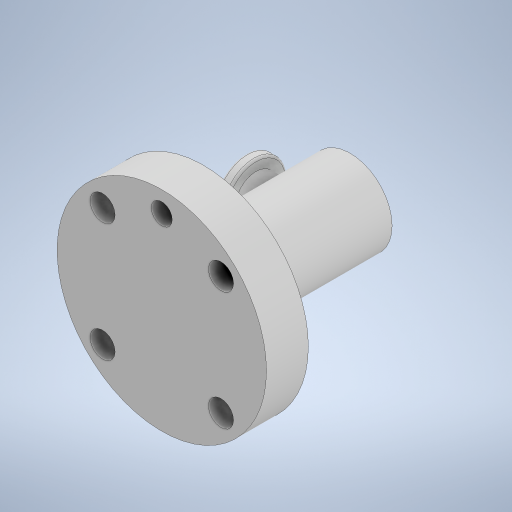
# Autodesk Inventor part: ACOPLE
Saved by Autodesk Inventor 2024 (Build 280153000, 153)
## iProperties
Created: 2023-05-11
Part Number: ACOPLE
Material: Genérico
Document SubType Name: Modeling
Designer: sebas
Density: 1 g/cm^3
Appearance: Valor por defecto
Author: sebas
Autodesk Inventor part; units mm, degrees
ref_plane "YZ Plane" through (0, 0, 0) normal (1, 0, 0) x (0, 1, 0)
ref_plane "XZ Plane" through (0, 0, 0) normal (0, 1, 0) x (-1, 0, 0)
sketch "Boceto4" plane through (0, 0, 0) normal (0, 0, 1) x (1, 0, 0)
  circle A0 centre (0, 0) radius 10
  circle A1 centre (0, 0) radius 7.582
  dimension "d6" = 20
  dimension "d7" = 15.164
  constraints: 2 centre point, 2 coincident
  measures "d6" diameter of A0
  measures "d7" diameter of A1
extrude "Extrusión3" add sketch "Boceto4" along normal blind 40
sketch "Boceto5" plane through (0, 0, 40) normal (0, 0, 1) x (1, 0, 0)
  circle A0 centre (0, 0) radius 7.582
  constraints: 1 centre point, 1 coincident
extrude "Extrusión4" add sketch "Boceto5" against normal blind 25
ref_plane "Plano de trabajo2" through (-10, 0, 0) normal (1, 0, 0) x (0, 1, 0)
sketch "Boceto6" plane through (-10, 0, 0) normal (1, 0, 0) x (0, 1, 0)
  line L0 (0, 0) -> (0, 10)
  circle A0 centre (0, 10) radius 5
  dimension "d14" = 10
  dimension "d15" = 10
  constraints: 2 end point, 1 centre point, 1 coincident, 1 vertical
  measures "d14" distance of L0.start L0.end
  measures "d15" diameter of A0
extrude "Extrusión5" cut sketch "Boceto6" along normal blind 10
ref_plane "Plano de trabajo3" through (-15, 0, 0) normal (1, 0, 0) x (0, 1, 0)
sketch "Boceto8" plane through (-15, 0, 0) normal (1, 0, 0) x (0, 1, 0)
  line L0 (0, 5) -> (0, 15)
  circle A0 centre (0, 10) radius 7.5
  circle A1 centre (0, 10) radius 2.5
  point P0 (0, 0)
  dimension "d21" = 15
  dimension "d22" = 5
  constraints: 2 centre point, 2 end point, 1 coincident, 1 midpoint, 1 vertical
  measures "d21" diameter of A0
  measures "d22" diameter of A1
extrude "Extrusión6" add sketch "Boceto8" along normal blind 2.5
fillet "Empalme1" radius 0.5 1 edges at (-15, -7.5, 10)
sketch "Boceto9" plane through (-10, 0, 0) normal (1, 0, 0) x (0, 1, 0)
  spline S0 degree 6 poles (0, 15) (-0.3834, 15) (-0.7632, 14.9647) (-1.1332, 14.8954) (-1.4876, 14.7952) (-1.821, 14.669) (-2.268, 14.4587) (-2.4027, 14.389) (-2.5328, 14.3156) (-2.6585, 14.2387) (-2.7797, 14.1586) (-3.056, 13.9622) (-3.2074, 13.8433) (-3.3509, 13.7196) (-3.4865, 13.5914) (-3.6147, 13.4594) (-3.888, 13.1522) (-4.0289, 12.9748) (-4.1583, 12.7923) (-4.2767, 12.6052) (-4.384, 12.414) (-4.5625, 12.0536) (-4.6367, 11.8855) (-4.7031, 11.7149) (-4.7617, 11.5423) (-4.8127, 11.3679) (-4.9038, 10.9965) (-4.9423, 10.7991) (-4.9711, 10.6003) (-4.9904, 10.4005) (-5, 10.2003) (-5, 9.6231) (-4.9659, 9.2469) (-4.898, 8.8739) (-4.7962, 8.5068) (-4.6605, 8.1486) (-4.3922, 7.6001) (-4.2815, 7.4015) (-4.159, 7.2074) (-4.0245, 7.0182) (-3.8778, 6.8346) (-3.5977, 6.5231) (-3.4697, 6.3924) (-3.3343, 6.2657) (-3.1912, 6.1433) (-3.0403, 6.0258) (-2.661, 5.7584) (-2.4247, 5.6131) (-2.1724, 5.48) (-1.9044, 5.3615) (-1.6213, 5.2601) (-1.1153, 5.1212) (-0.8996, 5.0736) (-0.6787, 5.0371) (-0.4539, 5.0124) (-0.2271, 5) (0, 5) knots 0 0 0 0 0 0 0 0.117694 0.117694 0.117694 0.117694 0.117694 0.170873 0.170873 0.170873 0.170873 0.170873 0.243512 0.243512 0.243512 0.243512 0.243512 0.33528 0.33528 0.33528 0.33528 0.33528 0.413125 0.413125 0.413125 0.413125 0.413125 0.499599 0.499599 0.499599 0.499599 0.499599 0.662325 0.662325 0.662325 0.662325 0.662325 0.757624 0.757624 0.757624 0.757624 0.757624 0.829819 0.829819 0.829819 0.829819 0.829819 0.929825 0.929825 0.929825 0.929825 0.929825 1 1 1 1 1 1 1 projected
  line L0 (0, 5) -> (0, 15)
  circle A0 centre (0, 10) radius 5
  point P0 (0, 0)
  point P1 (0, 15)
  constraints: 2 end point, 1 centre point, 1 midpoint, 1 vertical, 2 other
extrude "Extrusión7" add sketch "Boceto9" along normal blind 1.5 and the other way blind 2.5
fillet "Empalme2" radius 0.5 1 edges at (-12.5, -7.5, 10)
fillet "Empalme3" radius 0.5 1 edges at (-15, -2.5, 10)
sketch "Boceto10" plane through (-12.5, 0, 10) normal (-1, 0, 0) x (0, 0, 1)
  circle A0 centre (0, 0) radius 2.5
  point P0 (-10, 0)
  constraints: 1 centre point
extrude "Extrusión8" cut sketch "Boceto10" against normal blind 5
sketch "Boceto11" plane through (0, 0, 40) normal (0, 0, 1) x (1, 0, 0)
  circle A0 centre (0, 0) radius 25
  line L0 (0, 0) -> (49.3966, 0) construction
  line L1 (0, 0) -> (28.1488, 0) construction
  line L2 (0, 0) -> (14.1421, -14.1421)
  line L3 (14.1421, -14.1421) -> (14.1421, 14.1421)
  line L4 (0, 0) -> (14.1421, -14.1421)
  line L5 (0, 0) -> (14.1421, 14.1421)
  circle A1 centre (14.1421, 14.1421) radius 3
  circle A2 centre (14.1421, -14.1421) radius 3
  line L6 (0, 0) -> (0, -25)
  circle A3 centre (0, 0) radius 25
  line L7 (0, 0) -> (-49.3966, 0) construction
  line L8 (0, 0) -> (-28.1488, 0) construction
  line L9 (0, 0) -> (-14.1421, -14.1421)
  line L10 (-14.1421, -14.1421) -> (-14.1421, 14.1421)
  line L11 (0, 0) -> (-14.1421, -14.1421)
  line L12 (0, 0) -> (-14.1421, 14.1421)
  circle A4 centre (-14.1421, 14.1421) radius 3
  circle A5 centre (-14.1421, -14.1421) radius 3
  line L13 (0, 0) -> (0, 20)
  circle A6 centre (0, 20) radius 2.5
  dimension "d34" = 50
  dimension "d39" = 20
  dimension "d40" = 6
  dimension "d41" = 6
  dimension "d42" = 20
  dimension "d43" = 5
  constraints: 28 end point, 6 centre point, 6 coincident, 6 symmetric about line, 3 vertical, 2 horizontal, 1 line through centre, 1 vertical alignment, 4 other
  measures "d39" distance of L0.start L2.end
  measures "d40" diameter of A1
  measures "d41" diameter of A2
  measures "d42" distance of L0.start L13.end
  measures "d43" diameter of A6
extrude "Extrusión9" add sketch "Boceto11" along normal mid plane 10 contours A0 | L5 A1 L3 A2 L2 | L9 A5 L10 A4 L12
thread "Rosca1" size "M16x2" class "6H" standard "ISO Metric profile" full length
